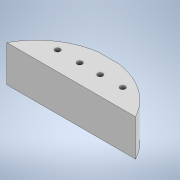
# Autodesk Inventor part: QuarterWheel
Saved by Autodesk Inventor 2020 (Build 240168000, 168)
## iProperties
Created: 2021-03-22
Part Number: QuarterWheel
Material: Generic
Document SubType Name: Modeling
Designer: tdmp4
Density: 1 g/cm^3
Appearance: Default
Author: tdmp4
Autodesk Inventor part; units mm, degrees
ref_plane "YZ Plane" through (0, 0, 0) normal (1, 0, 0) x (0, 1, 0)
ref_plane "XZ Plane" through (0, 0, 0) normal (0, 1, 0) x (-1, 0, 0)
ref_plane "XY Plane" through (0, 0, 0) normal (0, 0, 1) x (1, 0, 0)
sketch "Sketch1" plane through (0, 0, 0) normal (0, 1, 0) x (-1, 0, 0)
  arc A0 (-44.6217, -24.2805) -> (44.6217, -24.2805) centre (0, 0) ccw
  line L0 (44.6217, -24.2805) -> (-44.6217, -24.2805)
  line L1 (7.1173, -50.299) -> (-7.1173, -50.299)
  circle A1 centre (-22.5848, -37.3909) radius 1.778
  circle A2 centre (-7.1173, -37.2897) radius 1.778
  circle A3 centre (7.1173, -37.2897) radius 1.778
  circle A4 centre (22.5848, -37.3909) radius 1.778
  dimension "d0" = 101.6
  dimension "d1" = 3.556
  dimension "d2" = 3.556
  dimension "d3" = 3.556
  dimension "d4" = 3.556
  constraints: 5 centre point, 4 end point, 4 point on circle, 1 coincident, 1 horizontal
  measures "d0" diameter of A0
  measures "d1" diameter of A1
  measures "d2" diameter of A2
  measures "d3" diameter of A3
  measures "d4" diameter of A4
extrude "Extrusion1" add sketch "Sketch1" along normal blind 25.4 contours L0 A0 L1
body "Solid1"
